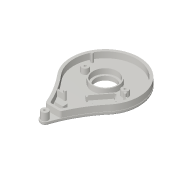
# Autodesk Inventor part: top
Saved by Autodesk Inventor 2016 SP1 (Build 200210100, 210)
## iProperties
Created: 2018-07-04
Part Number: top
Material: ABS-Kunststoff
Document SubType Name: Modeling
Designer: WhoTheHeck
Density: 1.06 g/cm^3
Appearance: Glatt - weiß
Author: WhoTheHeck
Autodesk Inventor part; units mm, degrees
ref_plane "YZ Plane" through (0, 0, 0) normal (1, 0, 0) x (0, 1, 0)
ref_plane "XZ Plane" through (0, 0, 0) normal (0, 1, 0) x (-1, 0, 0)
ref_plane "XY Plane" through (0, 0, 0) normal (0, 0, 1) x (1, 0, 0)
sketch "Skizze1" plane through (0, 0, 0) normal (0, 0, 1) x (1, 0, 0)
  circle A0 centre (0, 0) radius 13.65
  circle A1 centre (0, 0) radius 14.85
  line L0 (0, 0) -> (0, 14.85) construction
  line L1 (0, 0) -> (0, -28.15) construction
  circle A2 centre (0, -26.35) radius 1.8
  line L2 (0, -26.35) -> (0, -28.15) construction
  line L3 (-1.563745, -27.241461) -> (-12.900893, -7.354554)
  line L4 (12.900893, -7.354554) -> (1.563745, -27.241461)
  arc A3 (-1.705233, -26.926352) -> (-11.439829, -9.468517) centre (-53.809567, -44.537097) ccw
  arc A4 (11.439829, -9.468517) -> (1.705233, -26.926352) centre (53.809567, -44.537097) ccw
  line L5 (-6.539662, -18.513022) -> (-5.636186, -17.997968) construction
  dimension "d0" = 27.3
  dimension "d1" = 29.7
  dimension "d2" = 43
  dimension "d3" = 3.6
  dimension "d4" = 55
  dimension "d5" = 55
  dimension "d6" = 1.03998
  constraints: 15 point on circle, 12 end point, 8 tangent, 5 centre point, 2 coincident, 2 point on line, 2 vertical, 1 perpendicular
  measures "d0" diameter of A0
  measures "d1" diameter of A1
  measures "d2" distance of L1.end L0.end
  measures "d3" diameter of A2
  measures "d4" radius of A3
  measures "d5" radius of A4
  measures "d6" distance of L5.start L5.end
extrude "Extrusion1" add sketch "Skizze1" along normal blind 1.8 contours A0 | A1 | A1 A4 A2 A3 | A2
sketch "Skizze2" plane through (0, 0, 1.8) normal (0, 0, 1) x (1, 0, 0)
  circle A0 centre (0, 0) radius 4.25
  dimension "d9" = 8.5
  constraints: 1 centre point, 1 coincident
  measures "d9" diameter of A0
extrude "Extrusion2" cut sketch "Skizze2" against normal through all
sketch "Skizze3" plane through (0, 0, 1.8) normal (0, 0, 1) x (1, 0, 0)
  circle A0 centre (0, -26.35) radius 1.5
  line L0 (0, 0) -> (0, -28.167615) construction
  circle A1 centre (0, 0) radius 4.25 construction
  arc A2 (-1.705233, -26.926352) -> (1.705233, -26.926352) centre (0, -26.35) ccw construction
  arc A3 (11.439829, -9.468517) -> (1.705233, -26.926352) centre (53.809567, -44.537097) ccw construction
  arc A4 (11.439829, -9.468517) -> (-11.439829, -9.468517) centre (0, 0) ccw construction
  arc A5 (-1.705233, -26.926352) -> (-11.439829, -9.468517) centre (-53.809567, -44.537097) ccw construction
  circle A6 centre (0, -26.35) radius 0.5
  dimension "d12" = 3
  dimension "d13" = 1
  constraints: 2 centre point, 2 coincident, 2 end point, 1 vertical
  measures "d12" diameter of A0
  measures "d13" diameter of A6
extrude "Extrusion3" add sketch "Skizze3" along normal blind 3.2
sketch "Skizze4" plane through (0, 0, 1.8) normal (0, 0, 1) x (1, 0, 0)
  circle A0 centre (0, 0) radius 5.7
  circle A1 centre (0, 0) radius 5.2
  dimension "d16" = 11.4
  dimension "d17" = 10.4
  constraints: 2 centre point, 2 coincident
  measures "d16" diameter of A0
  measures "d17" diameter of A1
extrude "Extrusion4" add sketch "Skizze4" along normal blind 2.2
sketch "Skizze5" plane through (0, 0, 1.8) normal (0, 0, 1) x (1, 0, 0)
  line L0 (-13.330177, 0) -> (13.026214, 0) construction
  circle A0 centre (-8.7, 0) radius 1.5
  circle A1 centre (8.7, 0) radius 1.5
  circle A2 centre (8.7, 0) radius 0.5
  circle A3 centre (-8.7, 0) radius 0.5
  point P0 (0, 0)
  dimension "d20" = 3
  dimension "d21" = 3
  dimension "d22" = 1
  dimension "d23" = 1
  dimension "d24" = 17.4
  dimension "d25" = 8.7
  constraints: 4 centre point, 3 point on line, 2 coincident, 2 end point, 1 horizontal
  measures "d20" diameter of A0
  measures "d21" diameter of A1
  measures "d22" diameter of A2
  measures "d23" diameter of A3
  measures "d24" distance of A1.centre A0.centre
  measures "d25" distance of A0.centre point (0, 0)
extrude "Extrusion5" add sketch "Skizze5" along normal blind 2.4
sketch "Skizze6" plane through (0, 0, 1.8) normal (0, 0, 1) x (1, 0, 0)
  circle A0 centre (-8.7, 0) radius 1.5
  circle A1 centre (8.7, 0) radius 1.5
  circle A2 centre (0, -26.35) radius 1.5
  arc A3 (-1.705233, -26.926352) -> (1.705233, -26.926352) centre (0, -26.35) ccw
  arc A4 (11.439829, -9.468517) -> (1.705233, -26.926352) centre (53.809567, -44.537097) ccw
  arc A5 (11.439829, -9.468517) -> (-11.439829, -9.468517) centre (0, 0) ccw
  arc A6 (-1.705233, -26.926352) -> (-11.439829, -9.468517) centre (-53.809567, -44.537097) ccw
  circle A7 centre (0, 0) radius 5.7
  circle A8 centre (0, 0) radius 13.65
  line L0 (-2.3, -21.75) -> (2.3, -21.75)
  line L1 (0, 13.65) -> (0, -21.75) construction
  line L2 (0, -26.35) -> (0, -21.75) construction
  line L3 (0, 13.65) -> (0, 14.85) construction
  arc A9 (-1.705233, -26.926352) -> (-11.439829, -9.468517) centre (-53.809567, -44.537097) ccw construction
  arc A10 (-2.3, -21.75) -> (-10.436568, -8.797758) centre (-52.488674, -44.2466) ccw
  arc A11 (10.436568, -8.797758) -> (2.3, -21.75) centre (52.488674, -44.2466) ccw
  line L4 (-3.265825, -22.85) -> (3.265825, -22.85)
  dimension "d28" = 27.3
  dimension "d29" = 35.4
  dimension "d30" = 4.6
  dimension "d32" = 55
  dimension "d33" = 55
  dimension "d34" = 55
  dimension "d35" = 37.7
  constraints: 11 point on circle, 10 end point, 3 centre point, 2 horizontal, 2 midpoint, 2 tangent, 1 coincident, 1 collinear, 1 perpendicular, 1 point on line
  measures "d28" diameter of A8
  measures "d29" distance of L1.start L1.end
  measures "d30" distance of L0.start L0.end
  measures "d32" radius of A9
  measures "d33" radius of A10
  measures "d34" radius of A11
  measures "d35" distance from line of L3.end L4
extrude "Extrusion6" add sketch "Skizze6" along normal blind 2.6 contours A6 A5 A4 L4
fillet "Rundung1" radius 1 4 edges at (3.2658, -22.85, 3.1) (-3.2658, -22.85, 3.1) (-2.3, -21.75, 3.1) (2.3, -21.75, 3.1)
sketch "Skizze7" plane through (0, 0, 1.8) normal (0, 0, 1) x (1, 0, 0)
  arc A0 (-3.525237, -22.255127) -> (-2.610977, -22.85) centre (-2.610977, -21.85) ccw
  line L0 (-2.610977, -22.85) -> (2.610977, -22.85)
  arc A1 (2.610977, -22.85) -> (3.525237, -22.255127) centre (2.610977, -21.85) ccw
  arc A2 (11.439829, -9.468517) -> (3.525237, -22.255127) centre (53.809567, -44.537097) ccw
  arc A3 (11.439829, -9.468517) -> (-11.439829, -9.468517) centre (0, 0) ccw
  arc A4 (-3.525237, -22.255127) -> (-11.439829, -9.468517) centre (-53.809567, -44.537097) ccw
  arc A5 (10.436568, -8.797758) -> (-10.436568, -8.797758) centre (0, 0) ccw
  arc A6 (10.436568, -8.797758) -> (2.564219, -21.169582) centre (52.488674, -44.2466) ccw
  line L1 (1.656501, -21.75) -> (-1.656501, -21.75)
  arc A7 (-2.564219, -21.169582) -> (-10.436568, -8.797758) centre (-52.488674, -44.2466) ccw
  circle A8 centre (0, 0) radius 5.7
  circle A9 centre (8.7, 0) radius 1.5
  circle A10 centre (-8.7, 0) radius 1.5
  arc A11 (10.436568, -8.797758) -> (-10.436568, -8.797758) centre (0, 0) ccw
  arc A12 (-2.564219, -21.169582) -> (-10.436568, -8.797758) centre (-52.488674, -44.2466) ccw
  line L2 (-1.656501, -21.75) -> (1.656501, -21.75)
  arc A13 (10.436568, -8.797758) -> (2.564219, -21.169582) centre (52.488674, -44.2466) ccw
  circle A14 centre (-11, 5.3) radius 0.55
  circle A15 centre (11.5, -2.8) radius 0.55
  circle A16 centre (-2.65, -14.95) radius 0.55
  arc A17 (1.656501, -21.75) -> (2.564219, -21.169582) centre (1.656501, -20.75) ccw
  arc A18 (-2.564219, -21.169582) -> (-1.656501, -21.75) centre (-1.656501, -20.75) ccw
  arc A19 (1.656501, -21.75) -> (2.564219, -21.169582) centre (1.656501, -20.75) ccw
  arc A20 (-2.564219, -21.169582) -> (-1.656501, -21.75) centre (-1.656501, -20.75) ccw
  dimension "d40" = 1.1
  dimension "d41" = 1.1
  dimension "d42" = 1.1
  dimension "d43" = 6.8
  dimension "d44" = 2.65
  dimension "d45" = 2.8
  dimension "d46" = 2.8
  dimension "d47" = 5.3
  dimension "d48" = 2.3
  constraints: 3 centre point
  measures "d40" diameter of A14
  measures "d41" diameter of A15
  measures "d42" diameter of A16
  measures "d43" distance from line of A16.centre L2
  measures "d44" horizontal distance of point (0, 0) A16.centre
  measures "d45" horizontal distance of A15.centre A9.centre
  measures "d46" horizontal distance of A15.centre A9.centre
  measures "d47" vertical distance of A14.centre A10.centre
  measures "d48" horizontal distance of A10.centre A14.centre
extrude "Extrusion7" add sketch "Skizze7" along normal blind 3.7 contours A14 | A15 | A16
sketch "Skizze8" plane through (0, 0, 1.8) normal (0, 0, 1) x (1, 0, 0)
  circle A0 centre (11.5, -2.8) radius 0.55
  circle A1 centre (-11, 5.3) radius 0.55
  circle A2 centre (-2.65, -14.95) radius 0.55
  circle A3 centre (0, 0) radius 5.7
  circle A4 centre (8.7, 0) radius 1.5
  circle A5 centre (-8.7, 0) radius 1.5
  arc A6 (10.436568, -8.797758) -> (-10.436568, -8.797758) centre (0, 0) ccw
  arc A7 (-2.564219, -21.169582) -> (-10.436568, -8.797758) centre (-52.488674, -44.2466) ccw
  line L0 (-1.656501, -21.75) -> (1.656501, -21.75)
  arc A8 (10.436568, -8.797758) -> (2.564219, -21.169582) centre (52.488674, -44.2466) ccw
  line L1 (1.95, -20.45) -> (-1.95, -20.45)
  line L2 (-1.95, -20.45) -> (-1.95, -18.25)
  line L3 (-1.95, -18.25) -> (1.95, -18.25)
  line L4 (1.95, -18.25) -> (1.95, -20.45)
  line L5 (1.95, -20.45) -> (-1.95, -18.25) construction
  line L6 (-1.95, -20.45) -> (1.95, -18.25) construction
  line L7 (0, 13.65) -> (0, -19.35) construction
  arc A9 (1.656501, -21.75) -> (2.564219, -21.169582) centre (1.656501, -20.75) ccw
  arc A10 (-2.564219, -21.169582) -> (-1.656501, -21.75) centre (-1.656501, -20.75) ccw
  dimension "d51" = 3.9
  dimension "d52" = 2.2
  dimension "d53" = 33
  constraints: 14 end point, 2 midpoint, 2 parallel, 1 horizontal, 1 perpendicular, 1 point on circle, 1 vertical
  measures "d51" distance of L2.end L3.end
  measures "d52" distance of L3.end L1.start
  measures "d53" distance of L7.start L7.end
extrude "Extrusion8" add sketch "Skizze8" along normal up to surface (2.6 mm away) contours L1 L2 L3 L4
sketch "Skizze9" plane through (0, 0, 1.8) normal (0, 0, 1) x (1, 0, 0)
  line L0 (1.95, -18.25) -> (1.95, -20.45)
  line L1 (1.95, -20.45) -> (-1.95, -20.45)
  line L2 (-1.95, -20.45) -> (-1.95, -18.25)
  line L3 (-1.95, -18.25) -> (1.95, -18.25)
  circle A0 centre (11.5, -2.8) radius 0.55
  circle A1 centre (-11, 5.3) radius 0.55
  circle A2 centre (-2.65, -14.95) radius 0.55
  circle A3 centre (0, 0) radius 5.7
  circle A4 centre (8.7, 0) radius 1.5
  circle A5 centre (-8.7, 0) radius 1.5
  arc A6 (10.436568, -8.797758) -> (-10.436568, -8.797758) centre (0, 0) ccw
  arc A7 (-2.564219, -21.169582) -> (-10.436568, -8.797758) centre (-52.488674, -44.2466) ccw
  line L4 (-1.656501, -21.75) -> (1.656501, -21.75)
  arc A8 (10.436568, -8.797758) -> (2.564219, -21.169582) centre (52.488674, -44.2466) ccw
  line L5 (6.749028, -13.42804) -> (11.859018, -6.887551)
  line L6 (11.859018, -6.887551) -> (7.682561, -3.624545)
  line L7 (7.682561, -3.624545) -> (2.572571, -10.165034)
  line L8 (2.572571, -10.165034) -> (6.749028, -13.42804)
  line L9 (6.749028, -13.42804) -> (7.682561, -3.624545) construction
  line L10 (11.859018, -6.887551) -> (2.572571, -10.165034) construction
  circle A9 centre (11.5, -2.8) radius 0.55
  line L11 (11.5, -2.8) -> (9.653016, -5.164032) construction
  line L12 (2.572571, -10.165034) -> (2.178566, -9.857203)
  line L13 (2.178566, -9.857203) -> (7.288556, -3.316714)
  line L14 (7.288556, -3.316714) -> (7.682561, -3.624545)
  line L15 (7.288556, -3.316714) -> (7.596387, -2.922709)
  line L16 (7.596387, -2.922709) -> (12.053845, -6.405257)
  line L17 (2.178566, -9.857203) -> (1.790281, -10.354185)
  line L18 (1.790281, -10.354185) -> (2.814695, -11.154545)
  line L19 (2.814695, -11.154545) -> (3.20298, -10.657563)
  line L20 (5.882216, -12.750812) -> (5.469461, -13.279114)
  line L21 (5.469461, -13.279114) -> (6.498023, -14.082714)
  line L22 (6.749028, -13.42804) -> (6.870219, -13.522724)
  line L23 (11.22757, -8.043933) -> (10.191847, -7.234737)
  line L24 (10.191847, -7.234737) -> (10.561243, -6.76193)
  line L25 (10.561243, -6.76193) -> (11.596967, -7.571127)
  line L26 (11.596967, -7.571127) -> (11.22757, -8.043933)
  line L27 (11.22757, -8.043933) -> (10.561243, -6.76193) construction
  line L28 (10.191847, -7.234737) -> (11.596967, -7.571127) construction
  line L29 (9.334517, -10.371972) -> (8.344862, -9.598769)
  line L30 (8.344862, -9.598769) -> (8.714259, -9.125963)
  line L31 (8.714259, -9.125963) -> (9.703914, -9.899166)
  line L32 (9.703914, -9.899166) -> (9.334517, -10.371972)
  line L33 (9.334517, -10.371972) -> (8.714259, -9.125963) construction
  line L34 (8.344862, -9.598769) -> (9.703914, -9.899166) construction
  line L35 (7.493092, -12.740348) -> (6.497878, -11.962801)
  line L36 (6.497878, -11.962801) -> (6.867275, -11.489995)
  line L37 (6.867275, -11.489995) -> (7.862489, -12.267541)
  line L38 (7.862489, -12.267541) -> (7.493092, -12.740348)
  line L39 (7.493092, -12.740348) -> (6.867275, -11.489995) construction
  line L40 (6.497878, -11.962801) -> (7.862489, -12.267541) construction
  line L41 (11.859018, -6.887551) -> (12.053845, -6.405257)
  arc A10 (1.656501, -21.75) -> (2.564219, -21.169582) centre (1.656501, -20.75) ccw
  arc A11 (-2.564219, -21.169582) -> (-1.656501, -21.75) centre (-1.656501, -20.75) ccw
  point P0 (7.215795, -8.526292)
  point P1 (10.894407, -7.402932)
  point P2 (9.024388, -9.748967)
  point P3 (7.180183, -12.115171)
  dimension "d56" = 8.3
  dimension "d57" = 5.3
  dimension "d58" = 52
  dimension "d59" = 3
  dimension "d60" = 0.5
  dimension "d61" = 0.5
  dimension "d62" = 0.8
  dimension "d63" = 3.4
  dimension "d64" = 4.2
  dimension "d65" = 0.6
  dimension "d66" = 0.6
  dimension "d67" = 0.6
  dimension "d68" = 2.4
  dimension "d69" = 2.4
  dimension "d70" = 1
  constraints: 74 end point, 13 perpendicular, 10 parallel, 8 midpoint, 3 point on circle, 3 point on line, 2 collinear
  measures "d56" distance between parallel lines of L6 L8
  measures "d57" distance of L5.end L6.end
  measures "d58" angle of L3 L5
  measures "d59" distance of L11.start L11.end
  measures "d60" distance between parallel lines of L7 L13
  measures "d61" distance of L13.end L15.end
  measures "d62" distance between parallel lines of L7 L19
  measures "d63" distance between parallel lines of L19 L20
  measures "d64" distance between parallel lines of L7 L24
  measures "d65" distance of L23.end L24.end
  measures "d66" distance of L29.end L30.end
  measures "d67" distance of L35.end L36.end
  measures "d68" distance between parallel lines of L29 L37
  measures "d69" distance between parallel lines of L23 L31
  measures "d70" distance between parallel lines of L8 L35
extrude "Extrusion9" add sketch "Skizze9" along normal blind 2 contours L41 L6 A6 | A6 L6 L14 L15 L16 | L7 L12 L13 L14 | L25 L26 L23 A6 | A6 L23 L5 L25 | L5 L23 L24 L25 | L8 L19 L18 L17 L12 | L31 A8 L29 L5 | L5 L29 L30 L31 | L8 L22 A8 L21 L20 | L31 L32 L29 A8 | L37 A8 L35 L5 | L5 L35 L36 L37 | A8 L37 L38 L35
sketch "Skizze10" plane through (0, 0, 0) normal (0, 0, -1) x (-1, 0, 0)
  circle A0 centre (0, 0) radius 15
  circle A1 centre (0, 0) radius 4.25
  arc A2 (-1.705233, -26.926352) -> (1.705233, -26.926352) centre (0, -26.35) ccw
  arc A3 (11.439829, -9.468517) -> (1.705233, -26.926352) centre (53.809567, -44.537097) ccw
  arc A4 (11.439829, -9.468517) -> (-11.439829, -9.468517) centre (0, 0) ccw
  arc A5 (-1.705233, -26.926352) -> (-11.439829, -9.468517) centre (-53.809567, -44.537097) ccw
  circle A6 centre (0, -26.35) radius 0.5
  circle A7 centre (0, -26.35) radius 1.95
  arc A8 (-1.847031, -26.97528) -> (-11.559169, -9.559583) centre (-53.942787, -44.611385) ccw
  arc A9 (11.559169, -9.559583) -> (1.847031, -26.97528) centre (53.942787, -44.611385) ccw
  dimension "d73" = 30
  dimension "d74" = 3.9
  dimension "d75" = 1.8
  dimension "d76" = 55
  dimension "d77" = 55
  dimension "d78" = 55
  constraints: 8 point on circle, 4 centre point, 4 tangent, 2 coincident
  measures "d73" diameter of A0
  measures "d74" diameter of A7
  measures "d75" radius of A2
  measures "d76" radius of A5
  measures "d77" radius of A8
  measures "d78" radius of A9
sketch "Skizze10 outline for Extrusion10" plane through (0, 0, 0) normal (0, 0, -1) x (-1, 0, 0)
  arc A0 (-1.847031, -26.97528) -> (1.847031, -26.97528) centre (0, -26.35) ccw
  arc A1 (1.847031, -26.97528) -> (11.559169, -9.559583) centre (53.942787, -44.611385) cw
  arc A2 (11.559169, -9.559583) -> (-11.559169, -9.559583) centre (0, 0) ccw
  arc A3 (-11.559169, -9.559583) -> (-1.847031, -26.97528) centre (-53.942787, -44.611385) cw
  circle A4 centre (0, -26.35) radius 0.5
  circle A5 centre (0, 0) radius 4.25
extrude "Extrusion10" add sketch "Skizze10 outline for Extrusion10" against normal up to surface (1.8 mm away)
fillet "Rundung3" radius 1.5 4 edges at (5.9072, -17.8236, 0) (0, -28.3, 0) (-5.9072, -17.8236, 0) (0, 15, 0)
sketch "Skizze11" plane through (11.808081, -6.847754, 1.8) normal (-0.6156615, -0.7880108, 0) x (0.7880108, -0.6156615, 0)
  line L0 (0, 2) -> (0, 0)
  line L1 (-5.235359, 2) -> (0, 2)
  line L2 (-5.235359, 0) -> (-5.235359, 2)
  line L3 (0, 0) -> (-5.235359, 0)
  line L4 (-5.235359, 2) -> (0, 2)
  circle A0 centre (-3.089969, 2) radius 1.8
  point P0 (-13.520793, -1.8)
  dimension "d82" = 3.6
  constraints: 1 centre point, 1 point on line
  measures "d82" diameter of A0
extrude "Extrusion11" cut sketch "Skizze11" against normal up to surface (0.5 mm away) contours A0 L1 | L1 A0
fillet "Rundung4" radius 0.5 4 edges at (1.95, -20.45, 3.1) (1.95, -18.25, 3.1) (-1.95, -18.25, 3.1) (-1.95, -20.45, 3.1)
sketch "Skizze12" plane through (0, 0, 1.8) normal (0, 0, 1) x (1, 0, 0)
  line L0 (6.867275, -11.489995) -> (7.784673, -12.206745)
  arc A0 (9.225287, -10.286633) -> (7.784673, -12.206745) centre (52.488674, -44.2466) ccw
  line L1 (9.225287, -10.286633) -> (8.344862, -9.598769)
  line L2 (8.344862, -9.598769) -> (8.714259, -9.125963)
  line L3 (8.714259, -9.125963) -> (9.59834, -9.816682)
  arc A1 (10.436568, -8.797758) -> (9.59834, -9.816682) centre (52.488674, -44.2466) ccw
  arc A2 (10.436568, -8.797758) -> (11.100034, -7.94429) centre (0, 0) ccw
  line L4 (11.100034, -7.94429) -> (10.191847, -7.234737)
  line L5 (10.191847, -7.234737) -> (10.561243, -6.76193)
  line L6 (10.561243, -6.76193) -> (11.439099, -7.447786)
  arc A3 (11.439099, -7.447786) -> (11.808081, -6.847754) centre (0, 0) ccw
  line L7 (11.808081, -6.847754) -> (7.682561, -3.624545)
  line L8 (7.682561, -3.624545) -> (2.572571, -10.165034)
  line L9 (2.572571, -10.165034) -> (3.20298, -10.657563)
  line L10 (3.20298, -10.657563) -> (2.814695, -11.154545)
  line L11 (2.814695, -11.154545) -> (1.790281, -10.354185)
  line L12 (1.790281, -10.354185) -> (7.596387, -2.922709)
  line L13 (7.596387, -2.922709) -> (12.053845, -6.405257)
  arc A4 (12.053845, -6.405257) -> (-10.436568, -8.797758) centre (0, 0) ccw
  arc A5 (-2.564219, -21.169582) -> (-10.436568, -8.797758) centre (-52.488674, -44.2466) ccw
  arc A6 (-2.564219, -21.169582) -> (-1.656501, -21.75) centre (-1.656501, -20.75) ccw
  line L14 (-1.656501, -21.75) -> (1.656501, -21.75)
  arc A7 (1.656501, -21.75) -> (2.564219, -21.169582) centre (1.656501, -20.75) ccw
  arc A8 (6.498023, -14.082714) -> (2.564219, -21.169582) centre (52.488674, -44.2466) ccw
  line L15 (6.498023, -14.082714) -> (5.469461, -13.279114)
  line L16 (5.469461, -13.279114) -> (5.882216, -12.750812)
  line L17 (5.882216, -12.750812) -> (6.870219, -13.522724)
  arc A9 (7.437435, -12.696864) -> (6.870219, -13.522724) centre (52.488674, -44.2466) ccw
  line L18 (7.437435, -12.696864) -> (6.497878, -11.962801)
  line L19 (6.497878, -11.962801) -> (6.867275, -11.489995)
  line L20 (1.95, -18.75) -> (1.95, -19.95)
  arc A10 (1.45, -20.45) -> (1.95, -19.95) centre (1.45, -19.95) ccw
  line L21 (1.45, -20.45) -> (-1.45, -20.45)
  arc A11 (-1.95, -19.95) -> (-1.45, -20.45) centre (-1.45, -19.95) ccw
  line L22 (-1.95, -19.95) -> (-1.95, -18.75)
  arc A12 (-1.45, -18.25) -> (-1.95, -18.75) centre (-1.45, -18.75) ccw
  line L23 (-1.45, -18.25) -> (1.45, -18.25)
  arc A13 (1.95, -18.75) -> (1.45, -18.25) centre (1.45, -18.75) ccw
  circle A14 centre (11.5, -2.8) radius 0.55
  circle A15 centre (-11, 5.3) radius 0.55
  circle A16 centre (-2.65, -14.95) radius 0.55
  circle A17 centre (0, 0) radius 5.7
  circle A18 centre (8.7, 0) radius 1.5
  circle A19 centre (-8.7, 0) radius 1.5
  line L24 (-11.4748, 5.114129) -> (-12.58083, 5.653433)
  line L25 (-12.58083, 5.653433) -> (-12.317864, 6.192737)
  line L26 (-12.317864, 6.192737) -> (-11.211834, 5.653433)
  line L27 (-11.211834, 5.653433) -> (-11.4748, 5.114129)
  line L28 (-11.4748, 5.114129) -> (-12.317864, 6.192737) construction
  line L29 (-12.58083, 5.653433) -> (-11.211834, 5.653433) construction
  line L30 (9.304481, 0.3) -> (9.304481, -0.3)
  line L31 (-6.718455, -15.25) -> (-2.728073, -15.25)
  line L32 (-2.728073, -15.25) -> (-2.728073, -14.65)
  line L33 (-2.728073, -14.65) -> (-6.718455, -14.65)
  line L34 (-6.718455, -14.65) -> (-6.718455, -15.25)
  line L35 (-6.718455, -15.25) -> (-2.728073, -14.65) construction
  line L36 (-2.728073, -15.25) -> (-6.718455, -14.65) construction
  line L37 (11.71229, -2.539703) -> (13.656605, -3.165839)
  line L38 (13.656605, -3.165839) -> (13.472686, -3.736955)
  line L39 (13.472686, -3.736955) -> (11.528371, -3.110819)
  line L40 (11.528371, -3.110819) -> (11.71229, -2.539703)
  line L41 (11.71229, -2.539703) -> (13.472686, -3.736955) construction
  line L42 (13.656605, -3.165839) -> (11.528371, -3.110819) construction
  point P0 (-11.896332, 5.653433)
  point P1 (-4.723264, -14.95)
  point P2 (12.592488, -3.138329)
  dimension "d86" = 0.6
  dimension "d88" = 0.6
  dimension "d91" = 0.6
  constraints: 38 end point, 6 midpoint, 6 parallel, 4 perpendicular
  measures "d86" distance of L24.end L25.end
  measures "d88" distance of L32.end L31.end
  measures "d91" distance of L37.end L38.end
extrude "Extrusion12" add sketch "Skizze12" along normal blind 2.4 contours L31 L34 L33 A5 | A5 L33 A16 L31 | A16 L33 L32 L31 | L24 L25 L26 A4 | A4 L26 A15 L24 | A15 L26 L27 L24 | L37 L38 L39 A4 | A4 L39 A14 L37 | A14 L39 L40 L37 picked at (-2.884163, -14.971107) picked at (-11.409514, 5.387186) picked at (11.759324, -2.855993)
equation "\"d5\" = d4"
equation "\"d23\" = d22"
equation "\"d25\" = 0.5 * d24"
equation "\"d33\" = d32"
equation "\"d34\" = d33"
equation "\"d41\" = d40"
equation "\"d42\" = d41"
equation "\"d61\" = d60"
equation "\"d66\" = d65"
equation "\"d67\" = d66"
equation "\"d77\" = d76"
equation "\"d78\" = d77"
